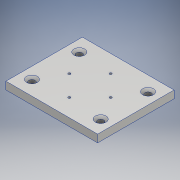
# Autodesk Inventor part: mounting_plate
Saved by Autodesk Inventor 2017 (Build 210142000, 142)
## iProperties
Created: 2017-09-27
Part Number: mounting_plate
Material: Aluminum 6061
Document SubType Name: Modeling
Designer: Thoma
Density: 2.7 g/cm^3
Appearance: Aluminum - Flat
Author: Thoma
Autodesk Inventor part; units mm, degrees
ref_plane "YZ Plane" through (0, 0, 0) normal (1, 0, 0) x (0, 1, 0)
ref_plane "XZ Plane" through (0, 0, 0) normal (0, 1, 0) x (-1, 0, 0)
ref_plane "XY Plane" through (0, 0, 0) normal (0, 0, 1) x (1, 0, 0)
sketch "Sketch1" plane through (0, 0, 0) normal (0, 0, 1) x (1, 0, 0)
  line L0 (0, 0) -> (120, 0)
  line L1 (120, 0) -> (120, 100)
  line L2 (120, 100) -> (0, 100)
  line L3 (0, 100) -> (0, 0)
  dimension "d0" = 120
  dimension "d1" = 100
  constraints: 8 end point, 2 parallel, 1 horizontal, 1 perpendicular
  measures "d0" distance of L2.end L1.end
  measures "d1" distance of L1.end L0.end
extrude "Extrusion1" add sketch "Sketch1" along normal blind 10
sketch "Sketch2" plane through (0, 0, 10) normal (0, 0, 1) x (1, 0, 0)
  line L0 (15, 19) -> (105, 19) construction
  line L1 (105, 19) -> (105, 81) construction
  line L2 (105, 81) -> (15, 81) construction
  line L3 (15, 81) -> (15, 19) construction
  circle A0 centre (60, 50) radius 8 construction
  line L4 (15, 19) -> (105, 81) construction
  line L5 (105, 19) -> (15, 81) construction
  point P0 (0, 0)
  dimension "d5" = 90
  dimension "d6" = 62
  constraints: 12 end point, 4 coincident, 2 midpoint, 2 parallel, 1 horizontal, 1 perpendicular
  measures "d5" distance of L2.end L1.end
  measures "d6" distance of L1.end L0.end
hole "Hole1" at (15, 81, 10) at (105, 81, 10) at (105, 19, 10) at (15, 19, 10) direction (0, 0, -1) diameter 8 end through all
chamfer "Chamfer1" distance 3 angle 45 1 edges at (15, 85, 10)
chamfer "Chamfer2" distance 3 angle 45 3 edges at (105, 85, 10) (105, 23, 10) (15, 23, 10)
sketch "Sketch3" plane through (0, 0, 0) normal (0, 0, -1) x (-1, 0, 0)
  circle A0 centre (-60, 50) radius 8 construction
  circle A1 centre (-60, 50) radius 27 construction
  point P0 (0, 0)
  point P1 (-60, 77)
  point P2 (-87, 50)
  point P3 (-60, 23)
  point P4 (-33, 50)
  dimension "d20" = 54
  dimension "d23" = 360
  constraints: 1 coincident, 1 vertical alignment, 7 other
hole "Hole2" at (60, 77, 0) at (87, 50, 0) at (60, 23, 0) at (33, 50, 0) direction (0, 0, 1) diameter 3 end through all
chamfer "Chamfer3" distance 2 angle 45 4 edges at (60, 75.5, 0) (33, 48.5, 0) (60, 21.5, 0) (87, 48.5, 0)
body "Solid1"
